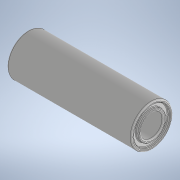
# Autodesk Inventor part: LM8LUU
Saved by Autodesk Inventor 2021 (Build 250183000, 183)
## iProperties
Created: 2016-03-22
Part Number: LM8LUU
Material: Типовые
Document SubType Name: Modeling
Designer: teacher
Density: 1 g/cm^3
Appearance: По умолчанию
Mass: 2.91864 g
Surface Area: 20.667 cm^2
Volume: 2.91864 cm^3
Author: teacher
Autodesk Inventor part; units mm, degrees
ref_plane "YZ Plane" through (0, 0, 0) normal (1, 0, 0) x (0, 1, 0)
ref_plane "XZ Plane" through (0, 0, 0) normal (0, 1, 0) x (-1, 0, 0)
ref_plane "XY Plane" through (0, 0, 0) normal (0, 0, 1) x (1, 0, 0)
sketch "Эскиз1" plane through (0, 0, 0) normal (1, 0, 0) x (0, 1, 0)
  circle A0 centre (0, 0) radius 7.5
  circle A1 centre (0, 0) radius 4
  dimension "d0" = 15
  dimension "d1" = 8
  constraints: 2 centre point, 2 coincident
  measures "d0" diameter of A0
  measures "d1" diameter of A1
extrude "Выдавливание1" add sketch "Эскиз1" along normal mid plane 45
sketch "Эскиз2" plane through (22.5, 0, 0) normal (1, 0, 0) x (0, 0, -1)
  circle A0 centre (0, 0) radius 5
  circle A1 centre (0, 0) radius 6.5
  dimension "d4" = 10
  dimension "d5" = 13
  constraints: 2 centre point, 2 coincident
  measures "d4" diameter of A0
  measures "d5" diameter of A1
extrude "Выдавливание2" cut sketch "Эскиз2" against normal blind 1
sketch "Эскиз3" plane through (-22.5, 0, 0) normal (-1, 0, 0) x (0, 0, 1)
  circle A0 centre (0, 0) radius 6.5
  circle A1 centre (0, 0) radius 5
  dimension "d9" = 13
  dimension "d10" = 10
  constraints: 2 centre point, 1 coincident
  measures "d9" diameter of A0
  measures "d10" diameter of A1
extrude "Выдавливание3" cut sketch "Эскиз3" against normal blind 1
fillet "Сопряжение1" radius 0.5 1 edges at (-22.5, -7.5, 0)
fillet "Сопряжение2" radius 0.5 3 edges at (-22.5, -4, 0) (22.5, -7.5, 0) (22.5, -4, 0)
chamfer "Фаска1" distance 0.2 angle 45 8 edges at (22.5, 0, 5) (22.5, 0, 6.5) (-22.5, 0, -5) (-22.5, 0, -6.5) (-21.5, 0, -5) (-21.5, 0, -6.5) (21.5, 0, 6.5) (21.5, 0, 5)
